Autodesk Fusion 360 part; units mm, degrees
(part 2 of 3)
sketch "Esquisse8" plane through (200, 0, 0) normal (1, 0, 0) x (0, 1, 0)
  line L0 (-239.4737, 3) -> (-239.4737, 6)
  line L1 (-239.4737, 6) -> (-228.9474, 6)
  line L2 (-228.9474, 6) -> (-228.9474, 3)
  line L3 (-228.9474, 3) -> (-218.4211, 3)
  line L4 (-218.4211, 3) -> (-218.4211, 6)
  line L5 (-218.4211, 6) -> (-207.8947, 6)
  line L6 (-207.8947, 6) -> (-207.8947, 3)
  line L7 (-207.8947, 3) -> (-197.3684, 3)
  line L8 (-197.3684, 3) -> (-197.3684, 6)
  line L9 (-197.3684, 6) -> (-186.8421, 6)
  line L10 (-186.8421, 6) -> (-186.8421, 3)
  line L11 (-186.8421, 3) -> (-176.3158, 3)
  line L12 (-176.3158, 3) -> (-176.3158, 6)
  line L13 (-176.3158, 6) -> (-165.7895, 6)
  line L14 (-165.7895, 6) -> (-165.7895, 3)
  line L15 (-165.7895, 3) -> (-155.2632, 3)
  line L16 (-155.2632, 3) -> (-155.2632, 6)
  line L17 (-155.2632, 6) -> (-144.7368, 6)
  line L18 (-144.7368, 6) -> (-144.7368, 3)
  line L19 (-144.7368, 3) -> (-134.2105, 3)
  line L20 (-134.2105, 3) -> (-134.2105, 6)
  line L21 (-134.2105, 6) -> (-123.6842, 6)
  line L22 (-123.6842, 6) -> (-123.6842, 3)
  line L23 (-123.6842, 3) -> (-113.1579, 3)
  line L24 (-113.1579, 3) -> (-113.1579, 6)
  line L25 (-113.1579, 6) -> (-102.6316, 6)
  line L26 (-102.6316, 6) -> (-102.6316, 3)
  line L27 (-102.6316, 3) -> (-92.1053, 3)
  line L28 (-92.1053, 3) -> (-92.1053, 6)
  line L29 (-92.1053, 6) -> (-81.5789, 6)
  line L30 (-81.5789, 6) -> (-81.5789, 3)
  line L31 (-81.5789, 3) -> (-71.0526, 3)
  line L32 (-71.0526, 3) -> (-71.0526, 6)
  line L33 (-71.0526, 6) -> (-60.5263, 6)
  line L34 (-60.5263, 6) -> (-60.5263, 3)
  line L35 (-60.5263, 3) -> (-50, 3)
  line L36 (-50, 3) -> (-50, 63)
  line L37 (-50, 63) -> (-250, 63)
  line L38 (-250, 63) -> (-250, 3)
  line L39 (-250, 3) -> (-239.4737, 3)
  line L40 (-250, 3) -> (-247, 3)
  line L41 (-247, 3) -> (-247, 15)
  line L42 (-247, 15) -> (-250, 15)
  line L43 (-250, 15) -> (-250, 3)
  line L44 (-53, 15) -> (-53, 3)
  line L45 (-53, 3) -> (-50, 3)
  line L46 (-50, 3) -> (-50, 15)
  line L47 (-50, 15) -> (-53, 15)
  line L48 (-250, 27) -> (-250, 15)
  line L49 (-250, 15) -> (-247, 15)
  line L50 (-247, 15) -> (-247, 27)
  line L51 (-247, 27) -> (-250, 27)
  line L52 (-53, 27) -> (-53, 15)
  line L53 (-53, 15) -> (-50, 15)
  line L54 (-50, 15) -> (-50, 27)
  line L55 (-50, 27) -> (-53, 27)
  line L56 (-250, 39) -> (-250, 27)
  line L57 (-250, 27) -> (-247, 27)
  line L58 (-247, 27) -> (-247, 39)
  line L59 (-247, 39) -> (-250, 39)
  line L60 (-53, 39) -> (-53, 27)
  line L61 (-53, 27) -> (-50, 27)
  line L62 (-50, 27) -> (-50, 39)
  line L63 (-50, 39) -> (-53, 39)
  line L64 (-250, 51) -> (-250, 39)
  line L65 (-250, 39) -> (-247, 39)
  line L66 (-247, 39) -> (-247, 51)
  line L67 (-247, 51) -> (-250, 51)
  line L68 (-53, 51) -> (-53, 39)
  line L69 (-53, 39) -> (-50, 39)
  line L70 (-50, 39) -> (-50, 51)
  line L71 (-50, 51) -> (-53, 51)
  line L72 (-250, 63) -> (-250, 51)
  line L73 (-250, 51) -> (-247, 51)
  line L74 (-247, 51) -> (-247, 63)
  line L75 (-247, 63) -> (-250, 63)
  line L76 (-53, 63) -> (-53, 51)
  line L77 (-53, 51) -> (-50, 51)
  line L78 (-50, 51) -> (-50, 63)
  line L79 (-50, 63) -> (-53, 63)
  dimension "d69" = 3
  dimension "d70" = 12
  dimension "d73" = 197
  dimension "d74" = 12
  constraint horizontal L40
  constraint vertical L41
  constraint horizontal L42
  constraint vertical L43
  constraint coincident L38.end L39.start
  measures "d69" distance of L38.end L40.end
  measures "d70" distance of L38.end L42.end
extrude "Extrusion7" cut sketch "Esquisse8" against normal blind 3 contours L38 L42 L48 L49 L50 L51 L57 | L38 L59 L64 L65 L66 L67 L73 | L36 L63 L68 L69 L70 L71 L77 | L36 L47 L52 L53 L54 L55 L61 bodies 7
sketch "Esquisse9" plane through (200, 0, 0) normal (1, 0, 0) x (0, 1, 0)
  line L0 (-53, 51) -> (-50, 51)
  line L1 (-50, 51) -> (-50, 63)
  line L2 (-50, 63) -> (-250, 63)
  line L3 (-250, 63) -> (-250, 51)
  line L4 (-250, 51) -> (-247, 51)
  line L5 (-247, 51) -> (-247, 39)
  line L6 (-247, 39) -> (-250, 39)
  line L7 (-250, 39) -> (-250, 27)
  line L8 (-250, 27) -> (-247, 27)
  line L9 (-247, 27) -> (-247, 15)
  line L10 (-247, 15) -> (-250, 15)
  line L11 (-250, 15) -> (-250, 3)
  line L12 (-250, 3) -> (-239.4737, 3)
  line L13 (-239.4737, 3) -> (-239.4737, 6)
  line L14 (-239.4737, 6) -> (-228.9474, 6)
  line L15 (-228.9474, 6) -> (-228.9474, 3)
  line L16 (-228.9474, 3) -> (-218.4211, 3)
  line L17 (-218.4211, 3) -> (-218.4211, 6)
  line L18 (-218.4211, 6) -> (-207.8947, 6)
  line L19 (-207.8947, 6) -> (-207.8947, 3)
  line L20 (-207.8947, 3) -> (-197.3684, 3)
  line L21 (-197.3684, 3) -> (-197.3684, 6)
  line L22 (-197.3684, 6) -> (-186.8421, 6)
  line L23 (-186.8421, 6) -> (-186.8421, 3)
  line L24 (-186.8421, 3) -> (-176.3158, 3)
  line L25 (-176.3158, 3) -> (-176.3158, 6)
  line L26 (-176.3158, 6) -> (-165.7895, 6)
  line L27 (-165.7895, 6) -> (-165.7895, 3)
  line L28 (-165.7895, 3) -> (-155.2632, 3)
  line L29 (-155.2632, 3) -> (-155.2632, 6)
  line L30 (-155.2632, 6) -> (-144.7368, 6)
  line L31 (-144.7368, 6) -> (-144.7368, 3)
  line L32 (-144.7368, 3) -> (-134.2105, 3)
  line L33 (-134.2105, 3) -> (-134.2105, 6)
  line L34 (-134.2105, 6) -> (-123.6842, 6)
  line L35 (-123.6842, 6) -> (-123.6842, 3)
  line L36 (-123.6842, 3) -> (-113.1579, 3)
  line L37 (-113.1579, 3) -> (-113.1579, 6)
  line L38 (-113.1579, 6) -> (-102.6316, 6)
  line L39 (-102.6316, 6) -> (-102.6316, 3)
  line L40 (-102.6316, 3) -> (-92.1053, 3)
  line L41 (-92.1053, 3) -> (-92.1053, 6)
  line L42 (-92.1053, 6) -> (-81.5789, 6)
  line L43 (-81.5789, 6) -> (-81.5789, 3)
  line L44 (-81.5789, 3) -> (-71.0526, 3)
  line L45 (-71.0526, 3) -> (-71.0526, 6)
  line L46 (-71.0526, 6) -> (-60.5263, 6)
  line L47 (-60.5263, 6) -> (-60.5263, 3)
  line L48 (-60.5263, 3) -> (-50, 3)
  line L49 (-50, 3) -> (-50, 15)
  line L50 (-50, 15) -> (-53, 15)
  line L51 (-53, 15) -> (-53, 27)
  line L52 (-53, 27) -> (-50, 27)
  line L53 (-50, 27) -> (-50, 39)
  line L54 (-50, 39) -> (-53, 39)
  line L55 (-53, 39) -> (-53, 51)
  line L56 (-250, 63) -> (-239.4737, 63)
  line L57 (-239.4737, 63) -> (-239.4737, 60)
  line L58 (-239.4737, 60) -> (-250, 60)
  line L59 (-250, 60) -> (-250, 63)
  line L60 (-228.9474, 60) -> (-239.4737, 60)
  line L61 (-239.4737, 60) -> (-239.4737, 63)
  line L62 (-239.4737, 63) -> (-228.9474, 63)
  line L63 (-228.9474, 63) -> (-228.9474, 60)
  line L64 (-218.4211, 60) -> (-228.9474, 60)
  line L65 (-228.9474, 60) -> (-228.9474, 63)
  line L66 (-228.9474, 63) -> (-218.4211, 63)
  line L67 (-218.4211, 63) -> (-218.4211, 60)
  line L68 (-207.8947, 60) -> (-218.4211, 60)
  line L69 (-218.4211, 60) -> (-218.4211, 63)
  line L70 (-218.4211, 63) -> (-207.8947, 63)
  line L71 (-207.8947, 63) -> (-207.8947, 60)
  line L72 (-197.3684, 60) -> (-207.8947, 60)
  line L73 (-207.8947, 60) -> (-207.8947, 63)
  line L74 (-207.8947, 63) -> (-197.3684, 63)
  line L75 (-197.3684, 63) -> (-197.3684, 60)
  line L76 (-186.8421, 60) -> (-197.3684, 60)
  line L77 (-197.3684, 60) -> (-197.3684, 63)
  line L78 (-197.3684, 63) -> (-186.8421, 63)
  line L79 (-186.8421, 63) -> (-186.8421, 60)
  line L80 (-176.3158, 60) -> (-186.8421, 60)
  line L81 (-186.8421, 60) -> (-186.8421, 63)
  line L82 (-186.8421, 63) -> (-176.3158, 63)
  line L83 (-176.3158, 63) -> (-176.3158, 60)
  line L84 (-165.7895, 60) -> (-176.3158, 60)
  line L85 (-176.3158, 60) -> (-176.3158, 63)
  line L86 (-176.3158, 63) -> (-165.7895, 63)
  line L87 (-165.7895, 63) -> (-165.7895, 60)
  line L88 (-155.2632, 60) -> (-165.7895, 60)
  line L89 (-165.7895, 60) -> (-165.7895, 63)
  line L90 (-165.7895, 63) -> (-155.2632, 63)
  line L91 (-155.2632, 63) -> (-155.2632, 60)
  line L92 (-144.7368, 60) -> (-155.2632, 60)
  line L93 (-155.2632, 60) -> (-155.2632, 63)
  line L94 (-155.2632, 63) -> (-144.7368, 63)
  line L95 (-144.7368, 63) -> (-144.7368, 60)
  line L96 (-134.2105, 60) -> (-144.7368, 60)
  line L97 (-144.7368, 60) -> (-144.7368, 63)
  line L98 (-144.7368, 63) -> (-134.2105, 63)
  line L99 (-134.2105, 63) -> (-134.2105, 60)
  line L100 (-123.6842, 60) -> (-134.2105, 60)
  line L101 (-134.2105, 60) -> (-134.2105, 63)
  line L102 (-134.2105, 63) -> (-123.6842, 63)
  line L103 (-123.6842, 63) -> (-123.6842, 60)
  line L104 (-113.1579, 60) -> (-123.6842, 60)
  line L105 (-123.6842, 60) -> (-123.6842, 63)
  line L106 (-123.6842, 63) -> (-113.1579, 63)
  line L107 (-113.1579, 63) -> (-113.1579, 60)
  line L108 (-102.6316, 60) -> (-113.1579, 60)
  line L109 (-113.1579, 60) -> (-113.1579, 63)
  line L110 (-113.1579, 63) -> (-102.6316, 63)
  line L111 (-102.6316, 63) -> (-102.6316, 60)
  line L112 (-92.1053, 60) -> (-102.6316, 60)
  line L113 (-102.6316, 60) -> (-102.6316, 63)
  line L114 (-102.6316, 63) -> (-92.1053, 63)
  line L115 (-92.1053, 63) -> (-92.1053, 60)
  line L116 (-81.5789, 60) -> (-92.1053, 60)
  line L117 (-92.1053, 60) -> (-92.1053, 63)
  line L118 (-92.1053, 63) -> (-81.5789, 63)
  line L119 (-81.5789, 63) -> (-81.5789, 60)
  line L120 (-71.0526, 60) -> (-81.5789, 60)
  line L121 (-81.5789, 60) -> (-81.5789, 63)
  line L122 (-81.5789, 63) -> (-71.0526, 63)
  line L123 (-71.0526, 63) -> (-71.0526, 60)
  line L124 (-60.5263, 60) -> (-71.0526, 60)
  line L125 (-71.0526, 60) -> (-71.0526, 63)
  line L126 (-71.0526, 63) -> (-60.5263, 63)
  line L127 (-60.5263, 63) -> (-60.5263, 60)
  line L128 (-50, 60) -> (-60.5263, 60)
  line L129 (-60.5263, 60) -> (-60.5263, 63)
  line L130 (-60.5263, 63) -> (-50, 63)
  line L131 (-50, 63) -> (-50, 60)
  dimension "d77" = 10.5263
  dimension "d78" = 3
  dimension "d81" = 10.5263
  dimension "d82" = 0
  constraint horizontal L56
  constraint vertical L57
  constraint horizontal L58
  constraint vertical L59
  constraint coincident L2.end L3.start
  measures "d77" distance of L2.end L56.end
  measures "d78" distance of L2.end L58.end
extrude "Extrusion8" cut sketch "Esquisse9" against normal blind 3 contours L2 L123 L124 L125 L126 L127 L129 | L2 L115 L116 L117 L118 L119 L121 | L2 L107 L108 L109 L110 L111 L113 | L2 L99 L100 L101 L102 L103 L105 | L2 L91 L92 L93 L94 L95 L97 | L2 L83 L84 L85 L86 L87 L89 | L2 L75 L76 L77 L78 L79 L81 | L2 L67 L68 L69 L70 L71 L73 | L2 L57 L60 L61 L62 L63 L65 bodies 7
ref_plane "Plan de construction6" through (100, -128.9474, 4.5) normal (1, 0, 0) x (0, 1, 0)
mirror "Symétrie miroir3" about plane through (100, -128.9474, 4.5) normal (1, 0, 0) of bodies 7 makes body 8
combine "Combiner4" operation cut target body 8 tool bodies 6 keep tools
ref_plane "Plan de construction7" through (121.0526, -250, 4.5) normal (0, -1, 0) x (1, 0, 0)
sketch "Esquisse10" plane through (0, -250, 0) normal (0, -1, 0) x (-1, 0, 0)
  line L0 (0, -3) -> (-200, -3)
  line L1 (-200, -3) -> (-200, -63)
  line L2 (-200, -63) -> (0, -63)
  line L3 (0, -63) -> (0, -3)
  point P0 (0, -3)
  point P1 (-200, -63)
  dimension "d88" = 200
  dimension "d89" = 60
  constraint horizontal L0
  constraint vertical L1
  constraint horizontal L2
  constraint vertical L3
  constraint coincident P0 L0.start
  measures "d88" distance of P0 L0.end
  measures "d89" distance of P0 L2.end
extrude "Extrusion9" add sketch "Esquisse10" against normal blind 3 separate body makes body 9
combine "Combiner5" operation cut target body 9 tool bodies 6 7 8 keep tools
sketch "Esquisse11" plane through (0, -250, 0) normal (0, -1, 0) x (1, 0, 0)
  line L0 (3, 63) -> (3, 51)
  line L1 (3, 51) -> (0, 51)
  line L2 (0, 51) -> (0, 39)
  line L3 (0, 39) -> (3, 39)
  line L4 (3, 39) -> (3, 27)
  line L5 (3, 27) -> (0, 27)
  line L6 (0, 27) -> (0, 15)
  line L7 (0, 15) -> (3, 15)
  line L8 (3, 15) -> (3, 3)
  line L9 (3, 3) -> (10.5263, 3)
  line L10 (10.5263, 3) -> (10.5263, 6)
  line L11 (10.5263, 6) -> (21.0526, 6)
  line L12 (21.0526, 6) -> (21.0526, 3)
  line L13 (21.0526, 3) -> (31.5789, 3)
  line L14 (31.5789, 3) -> (31.5789, 6)
  line L15 (31.5789, 6) -> (42.1053, 6)
  line L16 (42.1053, 6) -> (42.1053, 3)
  line L17 (42.1053, 3) -> (52.6316, 3)
  line L18 (52.6316, 3) -> (52.6316, 6)
  line L19 (52.6316, 6) -> (63.1579, 6)
  line L20 (63.1579, 6) -> (63.1579, 3)
  line L21 (63.1579, 3) -> (73.6842, 3)
  line L22 (73.6842, 3) -> (73.6842, 6)
  line L23 (73.6842, 6) -> (84.2105, 6)
  line L24 (84.2105, 6) -> (84.2105, 3)
  line L25 (84.2105, 3) -> (94.7368, 3)
  line L26 (94.7368, 3) -> (94.7368, 6)
  line L27 (94.7368, 6) -> (105.2632, 6)
  line L28 (105.2632, 6) -> (105.2632, 3)
  line L29 (105.2632, 3) -> (115.7895, 3)
  line L30 (115.7895, 3) -> (115.7895, 6)
  line L31 (115.7895, 6) -> (126.3158, 6)
  line L32 (126.3158, 6) -> (126.3158, 3)
  line L33 (126.3158, 3) -> (136.8421, 3)
  line L34 (136.8421, 3) -> (136.8421, 6)
  line L35 (136.8421, 6) -> (147.3684, 6)
  line L36 (147.3684, 6) -> (147.3684, 3)
  line L37 (147.3684, 3) -> (157.8947, 3)
  line L38 (157.8947, 3) -> (157.8947, 6)
  line L39 (157.8947, 6) -> (168.4211, 6)
  line L40 (168.4211, 6) -> (168.4211, 3)
  line L41 (168.4211, 3) -> (178.9474, 3)
  line L42 (178.9474, 3) -> (178.9474, 6)
  line L43 (178.9474, 6) -> (189.4737, 6)
  line L44 (189.4737, 6) -> (189.4737, 3)
  line L45 (189.4737, 3) -> (197, 3)
  line L46 (197, 3) -> (197, 15)
  line L47 (197, 15) -> (200, 15)
  line L48 (200, 15) -> (200, 27)
  line L49 (200, 27) -> (197, 27)
  line L50 (197, 27) -> (197, 39)
  line L51 (197, 39) -> (200, 39)
  line L52 (200, 39) -> (200, 51)
  line L53 (200, 51) -> (197, 51)
  line L54 (197, 51) -> (197, 63)
  line L55 (197, 63) -> (3, 63)
  line L56 (3, 63) -> (13.2105, 63)
  line L57 (13.2105, 63) -> (13.2105, 60)
  line L58 (13.2105, 60) -> (3, 60)
  line L59 (3, 60) -> (3, 63)
  line L60 (13.2105, 63) -> (23.4211, 63)
  line L61 (23.4211, 63) -> (23.4211, 60)
  line L62 (23.4211, 60) -> (13.2105, 60)
  line L63 (13.2105, 60) -> (13.2105, 63)
  line L64 (23.4211, 63) -> (33.6316, 63)
  line L65 (33.6316, 63) -> (33.6316, 60)
  line L66 (33.6316, 60) -> (23.4211, 60)
  line L67 (23.4211, 60) -> (23.4211, 63)
  line L68 (33.6316, 63) -> (43.8421, 63)
  line L69 (43.8421, 63) -> (43.8421, 60)
  line L70 (43.8421, 60) -> (33.6316, 60)
  line L71 (33.6316, 60) -> (33.6316, 63)
  line L72 (43.8421, 63) -> (54.0526, 63)
  line L73 (54.0526, 63) -> (54.0526, 60)
  line L74 (54.0526, 60) -> (43.8421, 60)
  line L75 (43.8421, 60) -> (43.8421, 63)
  line L76 (54.0526, 63) -> (64.2632, 63)
  line L77 (64.2632, 63) -> (64.2632, 60)
  line L78 (64.2632, 60) -> (54.0526, 60)
  line L79 (54.0526, 60) -> (54.0526, 63)
  line L80 (64.2632, 63) -> (74.4737, 63)
  line L81 (74.4737, 63) -> (74.4737, 60)
  line L82 (74.4737, 60) -> (64.2632, 60)
  line L83 (64.2632, 60) -> (64.2632, 63)
  line L84 (74.4737, 63) -> (84.6842, 63)
  line L85 (84.6842, 63) -> (84.6842, 60)
  line L86 (84.6842, 60) -> (74.4737, 60)
  line L87 (74.4737, 60) -> (74.4737, 63)
  line L88 (84.6842, 63) -> (94.8947, 63)
  line L89 (94.8947, 63) -> (94.8947, 60)
  line L90 (94.8947, 60) -> (84.6842, 60)
  line L91 (84.6842, 60) -> (84.6842, 63)
  line L92 (94.8947, 63) -> (105.1053, 63)
  line L93 (105.1053, 63) -> (105.1053, 60)
  line L94 (105.1053, 60) -> (94.8947, 60)
  line L95 (94.8947, 60) -> (94.8947, 63)
  line L96 (105.1053, 63) -> (115.3158, 63)
  line L97 (115.3158, 63) -> (115.3158, 60)
  line L98 (115.3158, 60) -> (105.1053, 60)
  line L99 (105.1053, 60) -> (105.1053, 63)
  line L100 (115.3158, 63) -> (125.5263, 63)
  line L101 (125.5263, 63) -> (125.5263, 60)
  line L102 (125.5263, 60) -> (115.3158, 60)
  line L103 (115.3158, 60) -> (115.3158, 63)
  line L104 (125.5263, 63) -> (135.7368, 63)
  line L105 (135.7368, 63) -> (135.7368, 60)
  line L106 (135.7368, 60) -> (125.5263, 60)
  line L107 (125.5263, 60) -> (125.5263, 63)
  line L108 (135.7368, 63) -> (145.9474, 63)
  line L109 (145.9474, 63) -> (145.9474, 60)
  line L110 (145.9474, 60) -> (135.7368, 60)
  line L111 (135.7368, 60) -> (135.7368, 63)
  line L112 (145.9474, 63) -> (156.1579, 63)
  line L113 (156.1579, 63) -> (156.1579, 60)
  line L114 (156.1579, 60) -> (145.9474, 60)
  line L115 (145.9474, 60) -> (145.9474, 63)
  line L116 (156.1579, 63) -> (166.3684, 63)
  line L117 (166.3684, 63) -> (166.3684, 60)
  line L118 (166.3684, 60) -> (156.1579, 60)
  line L119 (156.1579, 60) -> (156.1579, 63)
  line L120 (166.3684, 63) -> (176.5789, 63)
  line L121 (176.5789, 63) -> (176.5789, 60)
  line L122 (176.5789, 60) -> (166.3684, 60)
  line L123 (166.3684, 60) -> (166.3684, 63)
  line L124 (176.5789, 63) -> (186.7895, 63)
  line L125 (186.7895, 63) -> (186.7895, 60)
  line L126 (186.7895, 60) -> (176.5789, 60)
  line L127 (176.5789, 60) -> (176.5789, 63)
  line L128 (186.7895, 63) -> (197, 63)
  line L129 (197, 63) -> (197, 60)
  line L130 (197, 60) -> (186.7895, 60)
  line L131 (186.7895, 60) -> (186.7895, 63)
  dimension "d92" = 10.2105
  dimension "d93" = 3
  dimension "d96" = 10.2105
  dimension "d97" = 0
  constraint horizontal L56
  constraint vertical L57
  constraint horizontal L58
  constraint vertical L59
  constraint coincident L0.start L55.end
  measures "d92" distance of L0.start L56.end
  measures "d93" distance of L0.start L58.end
extrude "Extrusion10" cut sketch "Esquisse11" against normal blind 3 contours L55 L57 L60 L61 L62 L63 L67 | L55 L65 L68 L69 L70 L71 L75 | L55 L73 L76 L77 L78 L79 L83 | L55 L81 L84 L85 L86 L87 L91 | L55 L89 L92 L93 L94 L95 L99 | L55 L97 L100 L101 L102 L103 L107 | L55 L105 L108 L109 L110 L111 L115 | L55 L113 L116 L117 L118 L119 L123 | L55 L121 L124 L125 L126 L127 L131 bodies 9
ref_plane "Plan de construction8" through (100, -150, 4.5) normal (0, -1, 0) x (1, 0, 0)
mirror "Symétrie miroir4" about plane through (100, -150, 4.5) normal (0, -1, 0) of bodies 9 makes body 10
combine "Combiner6" operation cut target body 10 tool bodies 6 8 7 keep tools
ref_plane "Plan de construction9" through (191.8947, -248.5, 63) normal (0, 0, 1) x (1, 0, 0)
sketch "Esquisse12" plane through (0, 0, 63) normal (0, 0, 1) x (1, 0, 0)
  line L0 (200, -250) -> (0, -250)
  line L1 (0, -250) -> (0, -50)
  line L2 (0, -50) -> (200, -50)
  line L3 (200, -50) -> (200, -250)
  point P0 (200, -250)
  point P1 (0, -50)
  dimension "d103" = 200
  dimension "d104" = 200
  constraint horizontal L0
  constraint vertical L1
  constraint horizontal L2
  constraint vertical L3
  constraint coincident P0 L0.start
  measures "d103" distance of P0 L0.end
  measures "d104" distance of P0 L2.end
extrude "Extrusion11" add sketch "Esquisse12" against normal blind 3 separate body makes body 11
combine "Combiner7" operation cut target body 11 tool bodies 9 7 8 10 keep tools
sketch "Esquisse13" plane through (0, 200, 0) normal (0, 1, 0) x (-1, 0, 0)
  line L0 (-200, 57.7778) -> (-197, 57.7778)
  line L1 (-197, 57.7778) -> (-197, 43.3333)
  line L2 (-197, 43.3333) -> (-200, 43.3333)
  line L3 (-200, 43.3333) -> (-200, 28.8889)
  line L4 (-200, 28.8889) -> (-197, 28.8889)
  line L5 (-197, 28.8889) -> (-197, 14.4444)
  line L6 (-197, 14.4444) -> (-200, 14.4444)
  line L7 (-200, 14.4444) -> (-200, 0)
  line L8 (-200, 0) -> (-189.4737, 0)
  line L9 (-189.4737, 0) -> (-189.4737, 3)
  line L10 (-189.4737, 3) -> (-178.9474, 3)
  line L11 (-178.9474, 3) -> (-178.9474, 0)
  line L12 (-178.9474, 0) -> (-168.4211, 0)
  line L13 (-168.4211, 0) -> (-168.4211, 3)
  line L14 (-168.4211, 3) -> (-157.8947, 3)
  line L15 (-157.8947, 3) -> (-157.8947, 0)
  line L16 (-157.8947, 0) -> (-147.3684, 0)
  line L17 (-147.3684, 0) -> (-147.3684, 3)
  line L18 (-147.3684, 3) -> (-136.8421, 3)
  line L19 (-136.8421, 3) -> (-136.8421, 0)
  line L20 (-136.8421, 0) -> (-126.3158, 0)
  line L21 (-126.3158, 0) -> (-126.3158, 3)
  line L22 (-126.3158, 3) -> (-115.7895, 3)
  line L23 (-115.7895, 3) -> (-115.7895, 0)
  line L24 (-115.7895, 0) -> (-105.2632, 0)
  line L25 (-105.2632, 0) -> (-105.2632, 3)
  line L26 (-105.2632, 3) -> (-94.7368, 3)
  line L27 (-94.7368, 3) -> (-94.7368, 0)
  line L28 (-94.7368, 0) -> (-84.2105, 0)
  line L29 (-84.2105, 0) -> (-84.2105, 3)
  line L30 (-84.2105, 3) -> (-73.6842, 3)
  line L31 (-73.6842, 3) -> (-73.6842, 0)
  line L32 (-73.6842, 0) -> (-63.1579, 0)
  line L33 (-63.1579, 0) -> (-63.1579, 3)
  line L34 (-63.1579, 3) -> (-52.6316, 3)
  line L35 (-52.6316, 3) -> (-52.6316, 0)
  line L36 (-52.6316, 0) -> (-42.1053, 0)
  line L37 (-42.1053, 0) -> (-42.1053, 3)
  line L38 (-42.1053, 3) -> (-31.5789, 3)
  line L39 (-31.5789, 3) -> (-31.5789, 0)
  line L40 (-31.5789, 0) -> (-21.0526, 0)
  line L41 (-21.0526, 0) -> (-21.0526, 3)
  line L42 (-21.0526, 3) -> (-10.5263, 3)
  line L43 (-10.5263, 3) -> (-10.5263, 0)
  line L44 (-10.5263, 0) -> (0, 0)
  line L45 (0, 0) -> (0, 14.4444)
  line L46 (0, 14.4444) -> (-3, 14.4444)
  line L47 (-3, 14.4444) -> (-3, 28.8889)
  line L48 (-3, 28.8889) -> (0, 28.8889)
  line L49 (0, 28.8889) -> (0, 43.3333)
  line L50 (0, 43.3333) -> (-3, 43.3333)
  line L51 (-3, 43.3333) -> (-3, 57.7778)
  line L52 (-3, 57.7778) -> (0, 57.7778)
  line L53 (0, 57.7778) -> (0, 72.2222)
  line L54 (0, 72.2222) -> (-3, 72.2222)
  line L55 (-3, 72.2222) -> (-3, 86.6667)
  line L56 (-3, 86.6667) -> (0, 86.6667)
  line L57 (0, 86.6667) -> (0, 101.1111)
  line L58 (0, 101.1111) -> (-3, 101.1111)
  line L59 (-3, 101.1111) -> (-3, 115.5556)
  line L60 (-3, 115.5556) -> (0, 115.5556)
  line L61 (0, 115.5556) -> (0, 130)
  line L62 (0, 130) -> (-200, 130)
  line L63 (-200, 130) -> (-200, 115.5556)
  line L64 (-200, 115.5556) -> (-197, 115.5556)
  line L65 (-197, 115.5556) -> (-197, 101.1111)
  line L66 (-197, 101.1111) -> (-200, 101.1111)
  line L67 (-200, 101.1111) -> (-200, 86.6667)
  line L68 (-200, 86.6667) -> (-197, 86.6667)
  line L69 (-197, 86.6667) -> (-197, 72.2222)
  line L70 (-197, 72.2222) -> (-200, 72.2222)
  line L71 (-200, 72.2222) -> (-200, 57.7778)
  line L72 (-86, 79) -> (-114, 79)
  line L73 (-114, 79) -> (-114, 51)
  line L74 (-114, 51) -> (-86, 51)
  line L75 (-86, 51) -> (-86, 79)
  line L76 (-75, 25) -> (-126, 25)
  line L77 (-126, 25) -> (-126, 36)
  line L78 (-126, 36) -> (-75, 36)
  line L79 (-75, 36) -> (-75, 25)
extrude "Extrusion12" cut sketch "Esquisse13" against normal blind 3 contours L72 L73 L74 L75 | L76 L77 L78 L79 bodies 3
move_body "Déplacer1" bodies 6 7 8 10 9 to x (1, 0, 0) y (0, 1, 0) z (0, 0, 1) at (0, -180, 0)
sketch "Esquisse14" plane through (0, 0, 0) normal (0, -1, 0) x (1, 0, 0)
  line L0 (197, 57.7778) -> (200, 57.7778)
  line L1 (200, 57.7778) -> (200, 72.2222)
  line L2 (200, 72.2222) -> (197, 72.2222)
  line L3 (197, 72.2222) -> (197, 86.6667)
  line L4 (197, 86.6667) -> (200, 86.6667)
  line L5 (200, 86.6667) -> (200, 101.1111)
  line L6 (200, 101.1111) -> (197, 101.1111)
  line L7 (197, 101.1111) -> (197, 115.5556)
  line L8 (197, 115.5556) -> (200, 115.5556)
  line L9 (200, 115.5556) -> (200, 130)
  line L10 (200, 130) -> (0, 130)
  line L11 (0, 130) -> (0, 115.5556)
  line L12 (0, 115.5556) -> (3, 115.5556)
  line L13 (3, 115.5556) -> (3, 101.1111)
  line L14 (3, 101.1111) -> (0, 101.1111)
  line L15 (0, 101.1111) -> (0, 86.6667)
  line L16 (0, 86.6667) -> (3, 86.6667)
  line L17 (3, 86.6667) -> (3, 72.2222)
  line L18 (3, 72.2222) -> (0, 72.2222)
  line L19 (0, 72.2222) -> (0, 57.7778)
  line L20 (0, 57.7778) -> (3, 57.7778)
  line L21 (3, 57.7778) -> (3, 43.3333)
  line L22 (3, 43.3333) -> (0, 43.3333)
  line L23 (0, 43.3333) -> (0, 28.8889)
  line L24 (0, 28.8889) -> (3, 28.8889)
  line L25 (3, 28.8889) -> (3, 14.4444)
  line L26 (3, 14.4444) -> (0, 14.4444)
  line L27 (0, 14.4444) -> (0, 0)
  line L28 (0, 0) -> (10.5263, 0)
  line L29 (10.5263, 0) -> (10.5263, 3)
  line L30 (10.5263, 3) -> (21.0526, 3)
  line L31 (21.0526, 3) -> (21.0526, 0)
  line L32 (21.0526, 0) -> (31.5789, 0)
  line L33 (31.5789, 0) -> (31.5789, 3)
  line L34 (31.5789, 3) -> (42.1053, 3)
  line L35 (42.1053, 3) -> (42.1053, 0)
  line L36 (42.1053, 0) -> (52.6316, 0)
  line L37 (52.6316, 0) -> (52.6316, 3)
  line L38 (52.6316, 3) -> (63.1579, 3)
  line L39 (63.1579, 3) -> (63.1579, 0)
  line L40 (63.1579, 0) -> (73.6842, 0)
  line L41 (73.6842, 0) -> (73.6842, 3)
  line L42 (73.6842, 3) -> (84.2105, 3)
  line L43 (84.2105, 3) -> (84.2105, 0)
  line L44 (84.2105, 0) -> (94.7368, 0)
  line L45 (94.7368, 0) -> (94.7368, 3)
  line L46 (94.7368, 3) -> (105.2632, 3)
  line L47 (105.2632, 3) -> (105.2632, 0)
  line L48 (105.2632, 0) -> (115.7895, 0)
  line L49 (115.7895, 0) -> (115.7895, 3)
  line L50 (115.7895, 3) -> (126.3158, 3)
  line L51 (126.3158, 3) -> (126.3158, 0)
  line L52 (126.3158, 0) -> (136.8421, 0)
  line L53 (136.8421, 0) -> (136.8421, 3)
  line L54 (136.8421, 3) -> (147.3684, 3)
  line L55 (147.3684, 3) -> (147.3684, 0)
  line L56 (147.3684, 0) -> (157.8947, 0)
  line L57 (157.8947, 0) -> (157.8947, 3)
  line L58 (157.8947, 3) -> (168.4211, 3)
  line L59 (168.4211, 3) -> (168.4211, 0)
  line L60 (168.4211, 0) -> (178.9474, 0)
  line L61 (178.9474, 0) -> (178.9474, 3)
  line L62 (178.9474, 3) -> (189.4737, 3)
  line L63 (189.4737, 3) -> (189.4737, 0)
  line L64 (189.4737, 0) -> (200, 0)
  line L65 (200, 0) -> (200, 14.4444)
  line L66 (200, 14.4444) -> (197, 14.4444)
  line L67 (197, 14.4444) -> (197, 28.8889)
  line L68 (197, 28.8889) -> (200, 28.8889)
  line L69 (200, 28.8889) -> (200, 43.3333)
  line L70 (200, 43.3333) -> (197, 43.3333)
  line L71 (197, 43.3333) -> (197, 57.7778)
  circle A0 centre (15, 15) radius 2.5
  circle A1 centre (21.6667, 15) radius 2.5
  circle A2 centre (28.3333, 15) radius 2.5
  circle A3 centre (35, 15) radius 2.5
  circle A4 centre (41.6667, 15) radius 2.5
  circle A5 centre (48.3333, 15) radius 2.5
  circle A6 centre (55, 15) radius 2.5
  circle A7 centre (61.6667, 15) radius 2.5
  circle A8 centre (68.3333, 15) radius 2.5
  circle A9 centre (75, 15) radius 2.5
  circle A10 centre (81.6667, 15) radius 2.5
  circle A11 centre (88.3333, 15) radius 2.5
  circle A12 centre (95, 15) radius 2.5
  circle A13 centre (101.6667, 15) radius 2.5
  circle A14 centre (108.3333, 15) radius 2.5
  circle A15 centre (115, 15) radius 2.5
  circle A16 centre (121.6667, 15) radius 2.5
  circle A17 centre (128.3333, 15) radius 2.5
  circle A18 centre (135, 15) radius 2.5
  circle A19 centre (141.6667, 15) radius 2.5
  circle A20 centre (148.3333, 15) radius 2.5
  circle A21 centre (155, 15) radius 2.5
  circle A22 centre (161.6667, 15) radius 2.5
  circle A23 centre (168.3333, 15) radius 2.5
  circle A24 centre (175, 15) radius 2.5
  circle A25 centre (15, 21.6667) radius 2.5
  circle A26 centre (21.6667, 21.6667) radius 2.5
  circle A27 centre (28.3333, 21.6667) radius 2.5
  circle A28 centre (35, 21.6667) radius 2.5
  circle A29 centre (41.6667, 21.6667) radius 2.5
  circle A30 centre (48.3333, 21.6667) radius 2.5
  circle A31 centre (55, 21.6667) radius 2.5
  circle A32 centre (61.6667, 21.6667) radius 2.5
  circle A33 centre (68.3333, 21.6667) radius 2.5
  circle A34 centre (75, 21.6667) radius 2.5
  circle A35 centre (81.6667, 21.6667) radius 2.5
  circle A36 centre (88.3333, 21.6667) radius 2.5
  circle A37 centre (95, 21.6667) radius 2.5
  circle A38 centre (101.6667, 21.6667) radius 2.5
  circle A39 centre (108.3333, 21.6667) radius 2.5
  circle A40 centre (115, 21.6667) radius 2.5
  circle A41 centre (121.6667, 21.6667) radius 2.5
  circle A42 centre (128.3333, 21.6667) radius 2.5
  circle A43 centre (135, 21.6667) radius 2.5
  circle A44 centre (141.6667, 21.6667) radius 2.5
  circle A45 centre (148.3333, 21.6667) radius 2.5
  circle A46 centre (155, 21.6667) radius 2.5
  circle A47 centre (161.6667, 21.6667) radius 2.5
  circle A48 centre (168.3333, 21.6667) radius 2.5
  circle A49 centre (175, 21.6667) radius 2.5
  circle A50 centre (15, 28.3333) radius 2.5
  circle A51 centre (21.6667, 28.3333) radius 2.5
  circle A52 centre (28.3333, 28.3333) radius 2.5
  circle A53 centre (35, 28.3333) radius 2.5
  circle A54 centre (41.6667, 28.3333) radius 2.5
  circle A55 centre (48.3333, 28.3333) radius 2.5
  circle A56 centre (55, 28.3333) radius 2.5
  circle A57 centre (61.6667, 28.3333) radius 2.5
  circle A58 centre (68.3333, 28.3333) radius 2.5
  circle A59 centre (75, 28.3333) radius 2.5
  circle A60 centre (81.6667, 28.3333) radius 2.5
  circle A61 centre (88.3333, 28.3333) radius 2.5
  circle A62 centre (95, 28.3333) radius 2.5
  circle A63 centre (101.6667, 28.3333) radius 2.5
  circle A64 centre (108.3333, 28.3333) radius 2.5
  circle A65 centre (115, 28.3333) radius 2.5
  circle A66 centre (121.6667, 28.3333) radius 2.5
  circle A67 centre (128.3333, 28.3333) radius 2.5
  circle A68 centre (135, 28.3333) radius 2.5
  circle A69 centre (141.6667, 28.3333) radius 2.5
  circle A70 centre (148.3333, 28.3333) radius 2.5
  circle A71 centre (155, 28.3333) radius 2.5
  circle A72 centre (161.6667, 28.3333) radius 2.5
  circle A73 centre (168.3333, 28.3333) radius 2.5
  circle A74 centre (175, 28.3333) radius 2.5
  circle A75 centre (15, 35) radius 2.5
  circle A76 centre (21.6667, 35) radius 2.5
  circle A77 centre (28.3333, 35) radius 2.5
  circle A78 centre (35, 35) radius 2.5
  circle A79 centre (41.6667, 35) radius 2.5
  circle A80 centre (48.3333, 35) radius 2.5
  circle A81 centre (55, 35) radius 2.5
  circle A82 centre (61.6667, 35) radius 2.5
  circle A83 centre (68.3333, 35) radius 2.5
  circle A84 centre (75, 35) radius 2.5
  circle A85 centre (81.6667, 35) radius 2.5
  circle A86 centre (88.3333, 35) radius 2.5
  circle A87 centre (95, 35) radius 2.5
  circle A88 centre (101.6667, 35) radius 2.5
  circle A89 centre (108.3333, 35) radius 2.5
  circle A90 centre (115, 35) radius 2.5
  circle A91 centre (121.6667, 35) radius 2.5
  circle A92 centre (128.3333, 35) radius 2.5
  circle A93 centre (135, 35) radius 2.5
  circle A94 centre (141.6667, 35) radius 2.5
  circle A95 centre (148.3333, 35) radius 2.5
  circle A96 centre (155, 35) radius 2.5
  circle A97 centre (161.6667, 35) radius 2.5
  circle A98 centre (168.3333, 35) radius 2.5
  circle A99 centre (175, 35) radius 2.5
  dimension "d121" = 5
  dimension "d124" = 160
  dimension "d125" = 20
  measures "d121" diameter of A0
extrude "Extrusion13" cut sketch "Esquisse14" against normal blind 3 contours A0 | A1 | A2 | A3 | A4 | A5 | A6 | A7 | A8 | A9 | A10 | A11 | A12 | A13 | A14 | A15 | A16 | A17 | A18 | A19 | A20 | A21 | A22 | A23 | A24 | A25 | A26 | A27 | A28 | A29 | A30 | A31 | A32 | A33 | A34 | A35 | A36 | A37 | A38 | A39 | A40 | A41 | A42 | A43 | A44 | A45 | A46 | A47 | A48 | A49 | A50 | A51 | A52 | A53 | A54 | A55 | A56 | A57 | A58 | A59 | A60 | A61 | A62 | A63 | A64 | A65 | A66 | A67 | A68 | A69 | A70 | A71 | A72 | A73 | A74 | A75 | A76 | A77 | A78 | A79 | A80 | A81 | A82 | A83 | A84 | A85 | A86 | A87 | A88 | A89 | A90 | A91 | A92 | A93 | A94 | A95 | A96 | A97 | A98 | A99 bodies 2
move_body "Déplacer2" bodies 11 to x (1, 0, 0) y (0, 1, 0) z (0, 0, 1) at (0, -180, 0)
sketch "Esquisse15" plane through (0, -430, 0) normal (0, -1, 0) x (1, 0, 0)
  line L0 (135.7368, 60) -> (135.7368, 63)
  line L1 (135.7368, 63) -> (125.5263, 63)
  line L2 (125.5263, 63) -> (125.5263, 60)
  line L3 (125.5263, 60) -> (115.3158, 60)
  line L4 (115.3158, 60) -> (115.3158, 63)
  line L5 (115.3158, 63) -> (105.1053, 63)
  line L6 (105.1053, 63) -> (105.1053, 60)
  line L7 (105.1053, 60) -> (94.8947, 60)
  line L8 (94.8947, 60) -> (94.8947, 63)
  line L9 (94.8947, 63) -> (84.6842, 63)
  line L10 (84.6842, 63) -> (84.6842, 60)
  line L11 (84.6842, 60) -> (74.4737, 60)
  line L12 (74.4737, 60) -> (74.4737, 63)
  line L13 (74.4737, 63) -> (64.2632, 63)
  line L14 (64.2632, 63) -> (64.2632, 60)
  line L15 (64.2632, 60) -> (54.0526, 60)
  line L16 (54.0526, 60) -> (54.0526, 63)
  line L17 (54.0526, 63) -> (43.8421, 63)
  line L18 (43.8421, 63) -> (43.8421, 60)
  line L19 (43.8421, 60) -> (33.6316, 60)
  line L20 (33.6316, 60) -> (33.6316, 63)
  line L21 (33.6316, 63) -> (23.4211, 63)
  line L22 (23.4211, 63) -> (23.4211, 60)
  line L23 (23.4211, 60) -> (13.2105, 60)
  line L24 (13.2105, 60) -> (13.2105, 63)
  line L25 (13.2105, 63) -> (3, 63)
  line L26 (3, 63) -> (3, 51)
  line L27 (3, 51) -> (0, 51)
  line L28 (0, 51) -> (0, 39)
  line L29 (0, 39) -> (3, 39)
  line L30 (3, 39) -> (3, 27)
  line L31 (3, 27) -> (0, 27)
  line L32 (0, 27) -> (0, 15)
  line L33 (0, 15) -> (3, 15)
  line L34 (3, 15) -> (3, 3)
  line L35 (3, 3) -> (10.5263, 3)
  line L36 (10.5263, 3) -> (10.5263, 6)
  line L37 (10.5263, 6) -> (21.0526, 6)
  line L38 (21.0526, 6) -> (21.0526, 3)
  line L39 (21.0526, 3) -> (31.5789, 3)
  line L40 (31.5789, 3) -> (31.5789, 6)
  line L41 (31.5789, 6) -> (42.1053, 6)
  line L42 (42.1053, 6) -> (42.1053, 3)
  line L43 (42.1053, 3) -> (52.6316, 3)
  line L44 (52.6316, 3) -> (52.6316, 6)
  line L45 (52.6316, 6) -> (63.1579, 6)
  line L46 (63.1579, 6) -> (63.1579, 3)
  line L47 (63.1579, 3) -> (73.6842, 3)
  line L48 (73.6842, 3) -> (73.6842, 6)
  line L49 (73.6842, 6) -> (84.2105, 6)
  line L50 (84.2105, 6) -> (84.2105, 3)
  line L51 (84.2105, 3) -> (94.7368, 3)
  line L52 (94.7368, 3) -> (94.7368, 6)
  line L53 (94.7368, 6) -> (105.2632, 6)
  line L54 (105.2632, 6) -> (105.2632, 3)
  line L55 (105.2632, 3) -> (115.7895, 3)
  line L56 (115.7895, 3) -> (115.7895, 6)
  line L57 (115.7895, 6) -> (126.3158, 6)
  line L58 (126.3158, 6) -> (126.3158, 3)
  line L59 (126.3158, 3) -> (136.8421, 3)
  line L60 (136.8421, 3) -> (136.8421, 6)
  line L61 (136.8421, 6) -> (147.3684, 6)
  line L62 (147.3684, 6) -> (147.3684, 3)
  line L63 (147.3684, 3) -> (157.8947, 3)
  line L64 (157.8947, 3) -> (157.8947, 6)
  line L65 (157.8947, 6) -> (168.4211, 6)
  line L66 (168.4211, 6) -> (168.4211, 3)
  line L67 (168.4211, 3) -> (178.9474, 3)
  line L68 (178.9474, 3) -> (178.9474, 6)
  line L69 (178.9474, 6) -> (189.4737, 6)
  line L70 (189.4737, 6) -> (189.4737, 3)
  line L71 (189.4737, 3) -> (197, 3)
  line L72 (197, 3) -> (197, 15)
  line L73 (197, 15) -> (200, 15)
  line L74 (200, 15) -> (200, 27)
  line L75 (200, 27) -> (197, 27)
  line L76 (197, 27) -> (197, 39)
  line L77 (197, 39) -> (200, 39)
  line L78 (200, 39) -> (200, 51)
  line L79 (200, 51) -> (197, 51)
  line L80 (197, 51) -> (197, 63)
  line L81 (197, 63) -> (186.7895, 63)
  line L82 (186.7895, 63) -> (186.7895, 60)
  line L83 (186.7895, 60) -> (176.5789, 60)
  line L84 (176.5789, 60) -> (176.5789, 63)
  line L85 (176.5789, 63) -> (166.3684, 63)
  line L86 (166.3684, 63) -> (166.3684, 60)
  line L87 (166.3684, 60) -> (156.1579, 60)
  line L88 (156.1579, 60) -> (156.1579, 63)
  line L89 (156.1579, 63) -> (145.9474, 63)
  line L90 (145.9474, 63) -> (145.9474, 60)
  line L91 (145.9474, 60) -> (135.7368, 60)
  circle A0 centre (10, 15) radius 2.5
  circle A1 centre (17.5, 15) radius 2.5
  circle A2 centre (25, 15) radius 2.5
  circle A3 centre (32.5, 15) radius 2.5
  circle A4 centre (40, 15) radius 2.5
  circle A5 centre (47.5, 15) radius 2.5
  circle A6 centre (55, 15) radius 2.5
  circle A7 centre (62.5, 15) radius 2.5
  circle A8 centre (70, 15) radius 2.5
  circle A9 centre (77.5, 15) radius 2.5
  circle A10 centre (85, 15) radius 2.5
  circle A11 centre (92.5, 15) radius 2.5
  circle A12 centre (100, 15) radius 2.5
  circle A13 centre (107.5, 15) radius 2.5
  circle A14 centre (115, 15) radius 2.5
  circle A15 centre (122.5, 15) radius 2.5
  circle A16 centre (130, 15) radius 2.5
  circle A17 centre (137.5, 15) radius 2.5
  circle A18 centre (145, 15) radius 2.5
  circle A19 centre (152.5, 15) radius 2.5
  circle A20 centre (160, 15) radius 2.5
  circle A21 centre (167.5, 15) radius 2.5
  circle A22 centre (175, 15) radius 2.5
  circle A23 centre (182.5, 15) radius 2.5
  circle A24 centre (190, 15) radius 2.5
  circle A25 centre (10, 30) radius 2.5
  circle A26 centre (17.5, 30) radius 2.5
  circle A27 centre (25, 30) radius 2.5
  circle A28 centre (32.5, 30) radius 2.5
  circle A29 centre (40, 30) radius 2.5
  circle A30 centre (47.5, 30) radius 2.5
  circle A31 centre (55, 30) radius 2.5
  circle A32 centre (62.5, 30) radius 2.5
  circle A33 centre (70, 30) radius 2.5
  circle A34 centre (77.5, 30) radius 2.5
  circle A35 centre (85, 30) radius 2.5
  circle A36 centre (92.5, 30) radius 2.5
  circle A37 centre (100, 30) radius 2.5
  circle A38 centre (107.5, 30) radius 2.5
  circle A39 centre (115, 30) radius 2.5
  circle A40 centre (122.5, 30) radius 2.5
  circle A41 centre (130, 30) radius 2.5
  circle A42 centre (137.5, 30) radius 2.5
  circle A43 centre (145, 30) radius 2.5
  circle A44 centre (152.5, 30) radius 2.5
  circle A45 centre (160, 30) radius 2.5
  circle A46 centre (167.5, 30) radius 2.5
  circle A47 centre (175, 30) radius 2.5
  circle A48 centre (182.5, 30) radius 2.5
  circle A49 centre (190, 30) radius 2.5
  circle A50 centre (10, 45) radius 2.5
  circle A51 centre (17.5, 45) radius 2.5
  circle A52 centre (25, 45) radius 2.5
  circle A53 centre (32.5, 45) radius 2.5
  circle A54 centre (40, 45) radius 2.5
  circle A55 centre (47.5, 45) radius 2.5
  circle A56 centre (55, 45) radius 2.5
  circle A57 centre (62.5, 45) radius 2.5
  circle A58 centre (70, 45) radius 2.5
  circle A59 centre (77.5, 45) radius 2.5
  circle A60 centre (85, 45) radius 2.5
  circle A61 centre (92.5, 45) radius 2.5
  circle A62 centre (100, 45) radius 2.5
  circle A63 centre (107.5, 45) radius 2.5
  circle A64 centre (115, 45) radius 2.5
  circle A65 centre (122.5, 45) radius 2.5
  circle A66 centre (130, 45) radius 2.5
  circle A67 centre (137.5, 45) radius 2.5
  circle A68 centre (145, 45) radius 2.5
  circle A69 centre (152.5, 45) radius 2.5
  circle A70 centre (160, 45) radius 2.5
  circle A71 centre (167.5, 45) radius 2.5
  circle A72 centre (175, 45) radius 2.5
  circle A73 centre (182.5, 45) radius 2.5
  circle A74 centre (190, 45) radius 2.5
  dimension "d128" = 5
  dimension "d131" = 180
  dimension "d132" = 30
  measures "d128" diameter of A0
extrude "Extrusion14" cut sketch "Esquisse15" against normal blind 3 contours A0 | A1 | A2 | A3 | A4 | A5 | A6 | A7 | A8 | A9 | A10 | A11 | A12 | A13 | A14 | A15 | A16 | A17 | A18 | A19 | A20 | A21 | A22 | A23 | A24 | A25 | A26 | A27 | A28 | A29 | A30 | A31 | A32 | A33 | A34 | A35 | A36 | A37 | A38 | A39 | A40 | A41 | A42 | A43 | A44 | A45 | A46 | A47 | A48 | A49 | A50 | A51 | A52 | A53 | A54 | A55 | A56 | A57 | A58 | A59 | A60 | A61 | A62 | A63 | A64 | A65 | A66 | A67 | A68 | A69 | A70 | A71 | A72 | A73 | A74 bodies 9
sketch "Esquisse16" plane through (0, 0, 6) normal (0, 0, 1) x (-1, 0, 0)
  line L0 (-10.5263, 430) -> (-21.0526, 430)
  line L1 (-21.0526, 430) -> (-21.0526, 427)
  line L2 (-21.0526, 427) -> (-31.5789, 427)
  line L3 (-31.5789, 427) -> (-31.5789, 430)
  line L4 (-31.5789, 430) -> (-42.1053, 430)
  line L5 (-42.1053, 430) -> (-42.1053, 427)
  line L6 (-42.1053, 427) -> (-52.6316, 427)
  line L7 (-52.6316, 427) -> (-52.6316, 430)
  line L8 (-52.6316, 430) -> (-63.1579, 430)
  line L9 (-63.1579, 430) -> (-63.1579, 427)
  line L10 (-63.1579, 427) -> (-73.6842, 427)
  line L11 (-73.6842, 427) -> (-73.6842, 430)
  line L12 (-73.6842, 430) -> (-84.2105, 430)
  line L13 (-84.2105, 430) -> (-84.2105, 427)
  line L14 (-84.2105, 427) -> (-94.7368, 427)
  line L15 (-94.7368, 427) -> (-94.7368, 430)
  line L16 (-94.7368, 430) -> (-105.2632, 430)
  line L17 (-105.2632, 430) -> (-105.2632, 427)
  line L18 (-105.2632, 427) -> (-115.7895, 427)
  line L19 (-115.7895, 427) -> (-115.7895, 430)
  line L20 (-115.7895, 430) -> (-126.3158, 430)
  line L21 (-126.3158, 430) -> (-126.3158, 427)
  line L22 (-126.3158, 427) -> (-136.8421, 427)
  line L23 (-136.8421, 427) -> (-136.8421, 430)
  line L24 (-136.8421, 430) -> (-147.3684, 430)
  line L25 (-147.3684, 430) -> (-147.3684, 427)
  line L26 (-147.3684, 427) -> (-157.8947, 427)
  line L27 (-157.8947, 427) -> (-157.8947, 430)
  line L28 (-157.8947, 430) -> (-168.4211, 430)
  line L29 (-168.4211, 430) -> (-168.4211, 427)
  line L30 (-168.4211, 427) -> (-178.9474, 427)
  line L31 (-178.9474, 427) -> (-178.9474, 430)
  line L32 (-178.9474, 430) -> (-189.4737, 430)
  line L33 (-189.4737, 430) -> (-189.4737, 427)
  line L34 (-189.4737, 427) -> (-197, 427)
  line L35 (-197, 427) -> (-197, 419.4737)
  line L36 (-197, 419.4737) -> (-200, 419.4737)
  line L37 (-200, 419.4737) -> (-200, 408.9474)
  line L38 (-200, 408.9474) -> (-197, 408.9474)
  line L39 (-197, 408.9474) -> (-197, 398.4211)
  line L40 (-197, 398.4211) -> (-200, 398.4211)
  line L41 (-200, 398.4211) -> (-200, 387.8947)
  line L42 (-200, 387.8947) -> (-197, 387.8947)
  line L43 (-197, 387.8947) -> (-197, 377.3684)
  line L44 (-197, 377.3684) -> (-200, 377.3684)
  line L45 (-200, 377.3684) -> (-200, 366.8421)
  line L46 (-200, 366.8421) -> (-197, 366.8421)
  line L47 (-197, 366.8421) -> (-197, 356.3158)
  line L48 (-197, 356.3158) -> (-200, 356.3158)
  line L49 (-200, 356.3158) -> (-200, 345.7895)
  line L50 (-200, 345.7895) -> (-197, 345.7895)
  line L51 (-197, 345.7895) -> (-197, 335.2632)
  line L52 (-197, 335.2632) -> (-200, 335.2632)
  line L53 (-200, 335.2632) -> (-200, 324.7368)
  line L54 (-200, 324.7368) -> (-197, 324.7368)
  line L55 (-197, 324.7368) -> (-197, 314.2105)
  line L56 (-197, 314.2105) -> (-200, 314.2105)
  line L57 (-200, 314.2105) -> (-200, 303.6842)
  line L58 (-200, 303.6842) -> (-197, 303.6842)
  line L59 (-197, 303.6842) -> (-197, 293.1579)
  line L60 (-197, 293.1579) -> (-200, 293.1579)
  line L61 (-200, 293.1579) -> (-200, 282.6316)
  line L62 (-200, 282.6316) -> (-197, 282.6316)
  line L63 (-197, 282.6316) -> (-197, 272.1053)
  line L64 (-197, 272.1053) -> (-200, 272.1053)
  line L65 (-200, 272.1053) -> (-200, 261.5789)
  line L66 (-200, 261.5789) -> (-197, 261.5789)
  line L67 (-197, 261.5789) -> (-197, 251.0526)
  line L68 (-197, 251.0526) -> (-200, 251.0526)
  line L69 (-200, 251.0526) -> (-200, 240.5263)
  line L70 (-200, 240.5263) -> (-197, 240.5263)
  line L71 (-197, 240.5263) -> (-197, 233)
  line L72 (-197, 233) -> (-189.4737, 233)
  line L73 (-189.4737, 233) -> (-189.4737, 230)
  line L74 (-189.4737, 230) -> (-178.9474, 230)
  line L75 (-178.9474, 230) -> (-178.9474, 233)
  line L76 (-178.9474, 233) -> (-168.4211, 233)
  line L77 (-168.4211, 233) -> (-168.4211, 230)
  line L78 (-168.4211, 230) -> (-157.8947, 230)
  line L79 (-157.8947, 230) -> (-157.8947, 233)
  line L80 (-157.8947, 233) -> (-147.3684, 233)
  line L81 (-147.3684, 233) -> (-147.3684, 230)
  line L82 (-147.3684, 230) -> (-136.8421, 230)
  line L83 (-136.8421, 230) -> (-136.8421, 233)
  line L84 (-136.8421, 233) -> (-126.3158, 233)
  line L85 (-126.3158, 233) -> (-126.3158, 230)
  line L86 (-126.3158, 230) -> (-115.7895, 230)
  line L87 (-115.7895, 230) -> (-115.7895, 233)
  line L88 (-115.7895, 233) -> (-105.2632, 233)
  line L89 (-105.2632, 233) -> (-105.2632, 230)
  line L90 (-105.2632, 230) -> (-94.7368, 230)
  line L91 (-94.7368, 230) -> (-94.7368, 233)
  line L92 (-94.7368, 233) -> (-84.2105, 233)
  line L93 (-84.2105, 233) -> (-84.2105, 230)
  line L94 (-84.2105, 230) -> (-73.6842, 230)
  line L95 (-73.6842, 230) -> (-73.6842, 233)
  line L96 (-73.6842, 233) -> (-63.1579, 233)
  line L97 (-63.1579, 233) -> (-63.1579, 230)
  line L98 (-63.1579, 230) -> (-52.6316, 230)
  line L99 (-52.6316, 230) -> (-52.6316, 233)
  line L100 (-52.6316, 233) -> (-42.1053, 233)
  line L101 (-42.1053, 233) -> (-42.1053, 230)
  line L102 (-42.1053, 230) -> (-31.5789, 230)
  line L103 (-31.5789, 230) -> (-31.5789, 233)
  line L104 (-31.5789, 233) -> (-21.0526, 233)
  line L105 (-21.0526, 233) -> (-21.0526, 230)
  line L106 (-21.0526, 230) -> (-10.5263, 230)
  line L107 (-10.5263, 230) -> (-10.5263, 233)
  line L108 (-10.5263, 233) -> (-3, 233)
  line L109 (-3, 233) -> (-3, 240.5263)
  line L110 (-3, 240.5263) -> (0, 240.5263)
  line L111 (0, 240.5263) -> (0, 251.0526)
  line L112 (0, 251.0526) -> (-3, 251.0526)
  line L113 (-3, 251.0526) -> (-3, 261.5789)
  line L114 (-3, 261.5789) -> (0, 261.5789)
  line L115 (0, 261.5789) -> (0, 272.1053)
  line L116 (0, 272.1053) -> (-3, 272.1053)
  line L117 (-3, 272.1053) -> (-3, 282.6316)
  line L118 (-3, 282.6316) -> (0, 282.6316)
  line L119 (0, 282.6316) -> (0, 293.1579)
  line L120 (0, 293.1579) -> (-3, 293.1579)
  line L121 (-3, 293.1579) -> (-3, 303.6842)
  line L122 (-3, 303.6842) -> (0, 303.6842)
  line L123 (0, 303.6842) -> (0, 314.2105)
  line L124 (0, 314.2105) -> (-3, 314.2105)
  line L125 (-3, 314.2105) -> (-3, 324.7368)
  line L126 (-3, 324.7368) -> (0, 324.7368)
  line L127 (0, 324.7368) -> (0, 335.2632)
  line L128 (0, 335.2632) -> (-3, 335.2632)
  line L129 (-3, 335.2632) -> (-3, 345.7895)
  line L130 (-3, 345.7895) -> (0, 345.7895)
  line L131 (0, 345.7895) -> (0, 356.3158)
  line L132 (0, 356.3158) -> (-3, 356.3158)
  line L133 (-3, 356.3158) -> (-3, 366.8421)
  line L134 (-3, 366.8421) -> (0, 366.8421)
  line L135 (0, 366.8421) -> (0, 377.3684)
  line L136 (0, 377.3684) -> (-3, 377.3684)
  line L137 (-3, 377.3684) -> (-3, 387.8947)
  line L138 (-3, 387.8947) -> (0, 387.8947)
  line L139 (0, 387.8947) -> (0, 398.4211)
  line L140 (0, 398.4211) -> (-3, 398.4211)
  line L141 (-3, 398.4211) -> (-3, 408.9474)
  line L142 (-3, 408.9474) -> (0, 408.9474)
  line L143 (0, 408.9474) -> (0, 419.4737)
  line L144 (0, 419.4737) -> (-3, 419.4737)
  line L145 (-3, 419.4737) -> (-3, 427)
  line L146 (-3, 427) -> (-10.5263, 427)
  line L147 (-10.5263, 427) -> (-10.5263, 430)
  circle A0 centre (-25, 255) radius 10
  circle A1 centre (-175, 255) radius 10
  circle A2 centre (-25, 405) radius 10
  circle A3 centre (-175, 405) radius 10
  dimension "d135" = 20
  dimension "d138" = -150
  dimension "d139" = 150
  measures "d135" diameter of A0
extrude "Extrusion15" cut sketch "Esquisse16" against normal blind 3 contours A0 | A1 | A2 | A3 bodies 6
move_body "Déplacer3" bodies 8 11 6 9 10 7 to x (1, 0, 0) y (0, 1, 0) z (0, 0, 1) at (0, 125, 0)